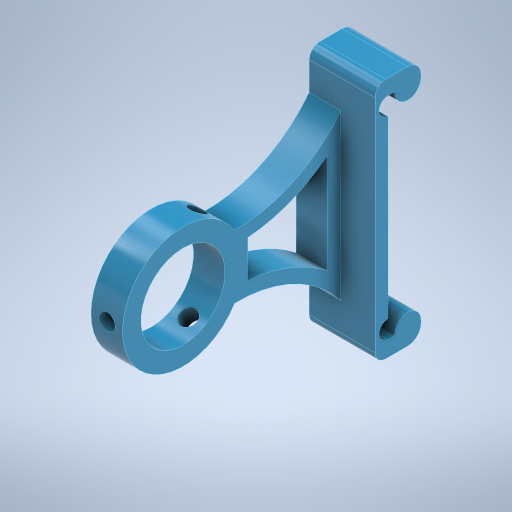
# Autodesk Inventor part: Rail-HeNeHolder
Saved by Autodesk Inventor 2023.1 (Build 271208000, 208)
## iProperties
Created: 2023-06-05
Part Number: Rail-HeNeHolder
Material: ABS Plastic
Document SubType Name: Modeling
Designer: hello
Density: 1.06 g/cm^3
Appearance: Sky Blue Dark
Mass: 24.8987 g
Surface Area: 148.331 cm^2
Volume: 23.4894 cm^3
Author: hello
Autodesk Inventor part; units mm, degrees
ref_plane "YZ Plane" through (0, 0, 0) normal (1, 0, 0) x (0, 1, 0)
ref_plane "XZ Plane" through (0, 0, 0) normal (0, 1, 0) x (-1, 0, 0)
sketch "Sketch1" plane through (0, 0, 0) normal (1, 0, 0) x (0, 1, 0)
  line L0 (-46, -7.5) -> (-46, 1)
  line L1 (-42, 5) -> (42, 5)
  line L2 (46, 1) -> (46, -7.5)
  line L3 (-41, -12.5) -> (-39.95, -12.5)
  line L4 (-40.25, -2.509) -> (-40.25, 0)
  line L5 (-40.25, 0) -> (40.25, 0)
  arc A0 (46, 1) -> (42, 5) centre (42, 1) ccw
  arc A1 (-42, 5) -> (-46, 1) centre (-42, 1) ccw
  arc A2 (40.25, 0) -> (33.25, 0) centre (36.75, 0) ccw
  arc A3 (-33.25, 0) -> (-40.25, 0) centre (-36.75, 0) ccw
  line L6 (40.25, 0) -> (40.25, -2.509)
  arc A4 (-39.95, -12.5) -> (-40.25, -2.509) centre (-39.95, -7.5) ccw
  arc A5 (-46, -7.5) -> (-41, -12.5) centre (-41, -7.5) ccw
  circle A6 centre (39.95, -7.5) radius 5
  line L7 (41, -12.5) -> (39.95, -12.5)
  arc A7 (41, -12.5) -> (46, -7.5) centre (41, -7.5) ccw
  circle A8 centre (0, 65) radius 16
  circle A9 centre (0, 65) radius 23
  arc A10 (-31.25, 5) -> (-12, 45.3786) centre (-61.9911, 44.4333) ccw
  arc A11 (12, 45.3786) -> (31.25, 5) centre (61.9911, 44.4333) ccw
  point P0 (0, 0)
  point P1 (-46, -12.5)
  point P2 (-46, 5)
  point P3 (46, 5)
  point P4 (46, -12.5)
  point P5 (0, 0)
  point P6 (-40.25, -1.2545)
  point P7 (40.25, -1.2545)
  point P8 (40.25, -2.509)
  point P9 (0, 5)
  dimension "d71" = 10
  dimension "d2" = 80.5
  dimension "d10" = 92
  dimension "d11" = 5
  dimension "d52" = 4
  dimension "d53" = 7
  dimension "d54" = 7
  dimension "d67" = 10
  dimension "d68" = 7.5
  dimension "d69" = 0.3
  dimension "d70" = 5
  dimension "d72" = 0.3
  dimension "d73" = 5
  dimension "d74" = 32
  dimension "d75" = 7
  dimension "d76" = 65
  dimension "d77" = 2
  dimension "d78" = 2
  dimension "d79" = 12
  dimension "d80" = 50
  constraints: 20 point on circle, 16 end point, 14 point on line, 11 centre point, 8 tangent, 4 midpoint, 4 vertical alignment, 3 horizontal alignment, 3 perpendicular, 2 equal radius, 2 horizontal, 2 vertical, 1 coincident, 3 other
  measures "d2" distance of L4.end L5.end
  measures "d10" distance of point (-46, 5) point (46, 5)
  measures "d11" distance between parallel lines of L1 L5
  measures "d52" radius of A0
  measures "d53" distance of A2.end L5.end
  measures "d54" distance of L4.end A3.start
  measures "d67" diameter of A4
  measures "d68" distance from line of L5 A4.centre
  measures "d69" distance from line of A4.centre L4
  measures "d70" radius of A5
  measures "d72" horizontal distance of point (39.95, -7.5) point (40.25, -1.255)
  measures "d73" radius of A7
  measures "d74" diameter of A8
  measures "d75" radial gap between concentric circles of A8 A9
  measures "d76" distance from line of L5 A8.centre
  measures "d77" horizontal distance of A10.start A3.start
  measures "d78" horizontal distance of A11.end A2.end
  measures "d79" horizontal distance of A9.start A8.centre
  measures "d80" radius of A10
extrude "Extrusion1" add sketch "Sketch1" along normal mid plane 12 contours L0 A1 L1 A0 L2 A7 L7 A6 L6 A2 L5 A3 L4 A4 L3 A5 | A10 A9 A11 L1 | A9 | A6
sketch "Sketch7" plane through (6, 0, 0) normal (1, 0, 0) x (0, 0, -1)
  arc A0 (-45.3786, 12) -> (-5, 31.25) centre (-44.4333, 61.9911) ccw projected
  arc A1 (-5, -31.25) -> (-45.3786, -12) centre (-44.4333, -61.9911) ccw projected
  arc A2 (-45.3786, 12) -> (-45.3786, -12) centre (-65, 0) ccw projected
  line L0 (-45.3786, 12) -> (-45.3786, -12)
  arc A3 (-45.3786, 12) -> (-5, 31.25) centre (-44.4333, 61.9911) ccw projected
  line L1 (-5, 31.25) -> (-5, -31.25)
  line L2 (0, -33.25) -> (0, 33.25) projected
  arc A4 (-45.3786, 12) -> (-5, 31.25) centre (-44.4333, 61.9911) ccw
  arc A5 (-5, -31.25) -> (-45.3786, -12) centre (-44.4333, -61.9911) ccw projected
  arc A6 (-5, -31.25) -> (-45.3786, -12) centre (-44.4333, -61.9911) ccw
  arc A7 (-10, -19.1035) -> (-40.3786, -7.1407) centre (-44.4333, -61.9911) ccw
  line L3 (-40.3786, -7.1407) -> (-40.3786, 7.1407)
  arc A8 (-40.3786, 7.1407) -> (-10, 19.1035) centre (-44.4333, 61.9911) ccw
  line L4 (-10, 19.1035) -> (-10, -19.1035)
  point P0 (0, 0)
  dimension "d81" = 5
  constraints: 10 point on circle, 8 end point, 4 centre point, 3 concentric, 2 point on line, 1 parallel, 1 vertical, 3 other
  measures "d81" distance between parallel lines of L0 L3
extrude "Extrusion4" cut sketch "Sketch7" against normal through all contours A7 L3 A8 L4
sketch "Sketch8" plane through (6, 0, 0) normal (1, 0, 0) x (0, 0, -1)
  line L0 (-40.3786, -7.1407) -> (-40.3786, 7.1407) projected
  arc A0 (-40.3786, 7.1407) -> (-10, 19.1035) centre (-44.4333, 61.9911) ccw projected
  line L1 (-10, 19.1035) -> (-10, -19.1035) projected
  arc A1 (-10, -19.1035) -> (-40.3786, -7.1407) centre (-44.4333, -61.9911) ccw projected
  arc A2 (0, -33.25) -> (0, -40.25) centre (0, -36.75) ccw projected
  line L2 (0, -33.25) -> (0, 33.25) projected
  arc A3 (0, 40.25) -> (0, 33.25) centre (0, 36.75) ccw projected
  line L3 (0, 40.25) -> (2.509, 40.25) projected
  arc A4 (2.509, 40.25) -> (12.5, 39.95) centre (7.5, 39.95) ccw projected
  line L4 (12.5, 39.95) -> (12.5, 41) projected
  arc A5 (12.5, 41) -> (7.5, 46) centre (7.5, 41) ccw projected
  line L5 (7.5, 46) -> (-1, 46) projected
  arc A6 (-1, 46) -> (-5, 42) centre (-1, 42) ccw projected
  line L6 (-5, 42) -> (-5, 31.25) projected
  arc A7 (-45.3786, 12) -> (-5, 31.25) centre (-44.4333, 61.9911) ccw projected
  arc A8 (-45.3786, 12) -> (-45.3786, -12) centre (-65, 0) ccw projected
  arc A9 (-5, -31.25) -> (-45.3786, -12) centre (-44.4333, -61.9911) ccw projected
  line L7 (-5, -31.25) -> (-5, -42) projected
  arc A10 (-5, -42) -> (-1, -46) centre (-1, -42) ccw projected
  line L8 (-1, -46) -> (7.5, -46) projected
  arc A11 (7.5, -46) -> (12.5, -41) centre (7.5, -41) ccw projected
  line L9 (12.5, -41) -> (12.5, -39.95) projected
  arc A12 (12.5, -39.95) -> (2.509, -40.25) centre (7.5, -39.95) ccw projected
  line L10 (2.509, -40.25) -> (0, -40.25) projected
  circle A13 centre (-65, 0) radius 16 projected
  line L11 (-5, 31.25) -> (-5, -31.25)
  point P0 (0, 0)
  constraints: 2 end point, 1 vertical
extrude "Extrusion5" add sketch "Sketch8" along normal blind 13 contours A2 L10 A12 L9 A11 L8 A10 L7 L11 L6 A6 L5 A5 L4 A4 L3 A3 L2
ref_plane "Work Plane1" through (0, 0, 88) normal (0, 0, 1) x (1, 0, 0)
sketch "Sketch9" plane through (0, 0, 88) normal (0, 0, 1) x (1, 0, 0)
  point P0 (0, 0)
  point P1 (0, 0)
  constraints: 1 coincident
hole "Hole4" at (0, 0, 88) direction (0, 0, -1) diameter 6.4 depth 10
pattern_circular "Circular Pattern1" count 3 over 360 about axis through (0, 0, 65) along (1, 0, 0) of "Hole4"
equation "\"d72\" = d69"
body "Solid1"
